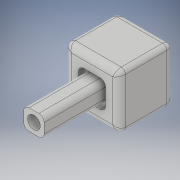
# Autodesk Inventor part: Square-Circle-Adapter V2D3
Saved by Autodesk Inventor 2017 (Build 210142000, 142)
## iProperties
Created: 2018-01-23
Part Number: Square-Circle-Adapter V2D3
Material: Generic
Document SubType Name: Modeling
Designer: Tripl_000
Density: 1 g/cm^3
Appearance: Default
Author: Tripl_000
Autodesk Inventor part; units mm, degrees
ref_plane "YZ Plane" through (0, 0, 0) normal (1, 0, 0) x (0, 1, 0)
ref_plane "XZ Plane" through (0, 0, 0) normal (0, 1, 0) x (-1, 0, 0)
ref_plane "XY Plane" through (0, 0, 0) normal (0, 0, 1) x (1, 0, 0)
sketch "Sketch1" plane through (0, 0, 0) normal (0, 0, 1) x (1, 0, 0)
  line L0 (-12.75, 12.75) -> (12.75, 12.75)
  line L1 (12.75, 12.75) -> (12.75, -12.75)
  line L2 (12.75, -12.75) -> (-12.75, -12.75)
  line L3 (-12.75, -12.75) -> (-12.75, 12.75)
  line L4 (-12.75, 12.75) -> (12.75, -12.75) construction
  line L5 (12.75, 12.75) -> (-12.75, -12.75) construction
  point P0 (0, 0)
  dimension "d0" = 25.5
  dimension "d1" = 25.5
  constraints: 12 end point, 2 midpoint, 2 parallel, 1 horizontal, 1 perpendicular
  measures "d0" distance of L0.start L0.end
  measures "d1" distance between parallel lines of L2 L0
extrude "Extrusion1" add sketch "Sketch1" along normal blind 25.4
sketch "Sketch2" plane through (0, 0, 25.4) normal (0, 0, 1) x (1, 0, 0)
  circle A0 centre (0, 0) radius 3
  dimension "d4" = 6
  constraints: 1 centre point, 1 coincident
  measures "d4" diameter of A0
extrude "Extrusion2" cut sketch "Sketch2" against normal through all
sketch "Sketch3" plane through (0, 0, 25.4) normal (0, 0, 1) x (1, 0, 0)
  line L0 (-6.4, 6.4) -> (6.4, 6.4)
  line L1 (6.4, 6.4) -> (6.4, -6.4)
  line L2 (6.4, -6.4) -> (-6.4, -6.4)
  line L3 (-6.4, -6.4) -> (-6.4, 6.4)
  line L4 (-6.4, 6.4) -> (6.4, -6.4) construction
  line L5 (6.4, 6.4) -> (-6.4, -6.4) construction
  point P0 (0, 0)
  dimension "d7" = 12.8
  dimension "d8" = 12.8
  constraints: 12 end point, 2 midpoint, 2 parallel, 1 horizontal, 1 perpendicular
  measures "d7" distance of L0.end L1.end
  measures "d8" distance of L0.start L0.end
extrude "Extrusion3" cut sketch "Sketch3" against normal blind 12.7
fillet "Fillet1" radius 2.5 4 edges at (6.4, 6.4, 19.05) (-6.4, 6.4, 19.05) (-6.4, -6.4, 19.05) (6.4, -6.4, 19.05)
fillet "Fillet2" radius 2 4 edges at (-12.75, 12.75, 12.7) (12.75, 12.75, 12.7) (-12.75, -12.75, 12.7) (12.75, -12.75, 12.7)
fillet "Fillet4" radius 3 8 edges at (12.1642, 12.1642, 0) (12.75, 0, 0) (12.1642, -12.1642, 0) (0, -12.75, 0) (-12.1642, -12.1642, 0) (-12.75, 0, 0) (-12.1642, 12.1642, 0) (0, 12.75, 0)
fillet "Fillet5" radius 3 8 edges at (12.1642, 12.1642, 25.4) (0, 12.75, 25.4) (-12.1642, 12.1642, 25.4) (-12.75, 0, 25.4) (-12.1642, -12.1642, 25.4) (0, -12.75, 25.4) (12.1642, -12.1642, 25.4) (12.75, 0, 25.4)
sketch "Sketch4" plane through (0, 0, 12.7) normal (0, 0, 1) x (1, 0, 0)
  line L0 (-4.8125, 4.8125) -> (4.8125, 4.8125)
  line L1 (4.8125, 4.8125) -> (4.8125, -4.8125)
  line L2 (4.8125, -4.8125) -> (-4.8125, -4.8125)
  line L3 (-4.8125, -4.8125) -> (-4.8125, 4.8125)
  line L4 (-4.8125, 4.8125) -> (4.8125, -4.8125) construction
  line L5 (4.8125, 4.8125) -> (-4.8125, -4.8125) construction
  line L6 (-3.9, 6.4) -> (3.9, 6.4) projected
  line L7 (6.4, 3.9) -> (6.4, -3.9) projected
  line L8 (-3.2125, 3.2125) -> (3.2125, 3.2125)
  line L9 (3.2125, 3.2125) -> (3.2125, -3.2125)
  line L10 (3.2125, -3.2125) -> (-3.2125, -3.2125)
  line L11 (-3.2125, -3.2125) -> (-3.2125, 3.2125)
  line L12 (-3.2125, 3.2125) -> (3.2125, -3.2125) construction
  line L13 (3.2125, 3.2125) -> (-3.2125, -3.2125) construction
  point P0 (0, 0)
  dimension "d17" = 1.5875
  dimension "d18" = 1.5875
  dimension "d19" = 1.6
  constraints: 24 end point, 4 midpoint, 4 parallel, 2 horizontal, 2 perpendicular, 1 point on line
  measures "d17" distance between parallel lines of L6 L0
  measures "d18" distance between parallel lines of L7 L1
  measures "d19" distance between parallel lines of L1 L9
extrude "Extrusion4" add sketch "Sketch4" along normal blind 40
fillet "Fillet7" radius 2.5 4 edges at (4.8125, 4.8125, 32.7) (4.8125, -4.8125, 32.7) (-4.8125, -4.8125, 32.7) (-4.8125, 4.8125, 32.7)
sketch "Sketch5" plane through (0, 0, 12.7) normal (0, 0, 1) x (1, 0, 0)
  circle A0 centre (0, 0) radius 3
  line L0 (-3.2125, -3.2125) -> (3.2125, -3.2125) projected
  line L1 (-3.2125, 3.2125) -> (3.2125, 3.2125)
  line L2 (3.2125, 3.2125) -> (3.2125, -3.2125)
  line L3 (3.2125, -3.2125) -> (-3.2125, -3.2125)
  line L4 (-3.2125, -3.2125) -> (-3.2125, 3.2125)
  line L5 (-3.2125, 3.2125) -> (3.2125, -3.2125) construction
  line L6 (3.2125, 3.2125) -> (-3.2125, -3.2125) construction
  constraints: 12 end point, 2 midpoint, 2 parallel, 1 centre point, 1 coincident, 1 horizontal, 1 perpendicular
extrude "Extrusion5" add sketch "Sketch5" along normal up to surface (40 mm away)
body "Solid1"
